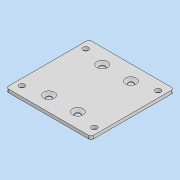
# Autodesk Inventor part: CCM_Mount_A
Saved by Autodesk Inventor 2020 (Build 240168000, 168)
## iProperties
Created: 2021-07-12
Part Number: CCM_Mount_A
Material: 一般
Document SubType Name: Modeling
Designer: magnarecta
Density: 1 g/cm^3
Appearance: 既定
Author: magnarecta
Autodesk Inventor part; units mm, degrees
ref_plane "YZ Plane" through (0, 0, 0) normal (1, 0, 0) x (0, 1, 0)
ref_plane "XZ Plane" through (0, 0, 0) normal (0, 1, 0) x (-1, 0, 0)
ref_plane "XY Plane" through (0, 0, 0) normal (0, 0, 1) x (1, 0, 0)
sketch "スケッチ1" plane through (0, 0, 0) normal (0, 1, 0) x (-1, 0, 0)
  line L0 (-40, -39) -> (40, -39)
  line L1 (40, -39) -> (40, 39)
  line L2 (40, 39) -> (-40, 39)
  line L3 (-40, 39) -> (-40, -39)
  line L4 (-40, -39) -> (40, 39) construction
  line L5 (40, -39) -> (-40, 39) construction
  point P0 (0, 0)
  dimension "d0" = 80
  dimension "d1" = 78
  constraints: 12 end point, 2 midpoint, 2 parallel, 1 horizontal, 1 perpendicular
  measures "d0" distance of L0.start L0.end
  measures "d1" distance of L0.end L1.end
extrude "押し出し1" add sketch "スケッチ1" along normal blind 3
sketch "スケッチ2" plane through (0, 3, 0) normal (0, 1, 0) x (1, 0, 0)
  line L0 (34, 30) -> (-34, 30)
  line L1 (-34, 30) -> (-34, -30)
  line L2 (-34, -30) -> (34, -30)
  line L3 (34, -30) -> (34, 30)
  line L4 (34, 30) -> (-34, -30) construction
  line L5 (-34, 30) -> (34, -30) construction
  point P0 (0, 0)
  dimension "d4" = 68
  dimension "d5" = 60
  constraints: 12 end point, 2 midpoint, 2 parallel, 1 horizontal, 1 perpendicular
  measures "d4" distance of L2.end L1.end
  measures "d5" distance of L1.end L0.end
hole "穴1" at (-34, 3, 30) at (34, 3, 30) at (34, 3, -30) at (-34, 3, -30) direction (0, -1, 0) diameter 5.2 depth 8 tip angle 118
sketch "スケッチ3" plane through (0, 3, 0) normal (0, 1, 0) x (1, 0, 0)
  line L0 (13.5, 25) -> (-13.5, 25)
  line L1 (-13.5, 25) -> (-13.5, -25)
  line L2 (-13.5, -25) -> (13.5, -25)
  line L3 (13.5, -25) -> (13.5, 25)
  line L4 (13.5, 25) -> (-13.5, -25) construction
  line L5 (-13.5, 25) -> (13.5, -25) construction
  point P0 (0, 0)
  dimension "d13" = 27
  dimension "d14" = 50
  constraints: 12 end point, 4 coincident, 2 midpoint, 2 parallel, 1 horizontal, 1 perpendicular
  measures "d13" distance of L0.start L0.end
  measures "d14" distance of L0.end L1.end
hole "穴2" at (-13.5, 3, 25) at (13.5, 3, 25) at (13.5, 3, -25) at (-13.5, 3, -25) direction (0, -1, 0) diameter 5.2 depth 8 tip angle 118 countersink diameter 10 countersink angle 90
fillet "フィレット2" radius 2 4 edges at (-40, 1.5, 39) (40, 1.5, 39) (40, 1.5, -39) (-40, 1.5, -39)
